Autodesk Inventor part; units mm, degrees
(part 2 of 2)
  spline S246 degree 2 poles (-6.4112, 55.0598) (-7.1438, 55.0598) (-8.0125, 55.9058) (-8.0125, 56.5866) knots 0 0 0 1 2 2 2
  spline S247 degree 2 poles (-8.0125, 56.5866) (-8.0125, 56.8945) (-7.8504, 57.3645) (-7.6786, 57.5428) knots 0 0 0 1 2 2 2
  spline S248 degree 2 poles (-7.6786, 57.5428) (-7.5068, 57.7211) (-7.0109, 57.9091) (-6.6511, 57.9091) knots 0 0 0 1 2 2 2
  line L247 (-6.6511, 57.9091) -> (-6.3755, 57.9091)
  line L248 (-6.3755, 57.9091) -> (-6.3755, 55.6238)
  spline S249 degree 2 poles (-6.3755, 55.6238) (-5.8537, 55.6238) (-5.2994, 56.2041) (-5.2994, 56.713) knots 0 0 0 1 2 2 2
  spline S250 degree 2 poles (-5.2994, 56.713) (-5.2994, 56.8977) (-5.3739, 57.2478) (-5.4323, 57.3905) knots 0 0 0 1 2 2 2
  spline S251 degree 2 poles (-5.4323, 57.3905) (-5.4971, 57.5396) (-5.6105, 57.747) (-5.6624, 57.8151) knots 0 0 0 1 2 2 2
  line L249 (-5.6624, 57.8151) -> (-5.6624, 57.8475)
  line L250 (-5.6624, 57.8475) -> (-5.1114, 57.8475)
  spline S252 degree 2 poles (-5.1114, 57.8475) (-5.0757, 57.7503) (-4.972, 57.4618) (-4.9428, 57.3451) knots 0 0 0 1 2 2 2
  spline S253 degree 2 poles (-4.9428, 57.3451) (-4.9007, 57.183) (-4.8585, 56.9204) (-4.8585, 56.7195) knots 0 0 0 1 2 2 2
  spline S254 degree 2 poles (-6.7613, 57.3678) (-6.9655, 57.3613) (-7.2637, 57.2673) (-7.3642, 57.1798) knots 0 0 0 1 2 2 2
  spline S255 degree 2 poles (-7.3642, 57.1798) (-7.4776, 57.0825) (-7.5976, 56.7778) (-7.5976, 56.5541) knots 0 0 0 1 2 2 2
  spline S256 degree 2 poles (-7.5976, 56.5541) (-7.5976, 56.3305) (-7.4776, 56.0225) (-7.361, 55.8961) knots 0 0 0 1 2 2 2
  spline S257 degree 2 poles (-7.361, 55.8961) (-7.241, 55.7729) (-6.9525, 55.64) (-6.7613, 55.6238) knots 0 0 0 1 2 2 2
  line L251 (-6.7613, 55.6238) -> (-6.7613, 57.3678)
  spline S258 degree 2 poles (-4.8585, 59.9026) (-4.8585, 59.1149) (-5.6657, 58.243) (-6.4112, 58.243) knots 0 0 0 1 2 2 2
  spline S259 degree 2 poles (-6.4112, 58.243) (-7.1438, 58.243) (-8.0125, 59.089) (-8.0125, 59.7697) knots 0 0 0 1 2 2 2
  spline S260 degree 2 poles (-8.0125, 59.7697) (-8.0125, 60.0776) (-7.8504, 60.5477) (-7.6786, 60.7259) knots 0 0 0 1 2 2 2
  spline S261 degree 2 poles (-7.6786, 60.7259) (-7.5068, 60.9042) (-7.0109, 61.0922) (-6.6511, 61.0922) knots 0 0 0 1 2 2 2
  line L252 (-6.6511, 61.0922) -> (-6.3755, 61.0922)
  line L253 (-6.3755, 61.0922) -> (-6.3755, 58.807)
  spline S262 degree 2 poles (-6.3755, 58.807) (-5.8537, 58.807) (-5.2994, 59.3872) (-5.2994, 59.8961) knots 0 0 0 1 2 2 2
  spline S263 degree 2 poles (-5.2994, 59.8961) (-5.2994, 60.0809) (-5.3739, 60.431) (-5.4323, 60.5736) knots 0 0 0 1 2 2 2
  spline S264 degree 2 poles (-5.4323, 60.5736) (-5.4971, 60.7227) (-5.6105, 60.9302) (-5.6624, 60.9982) knots 0 0 0 1 2 2 2
  line L254 (-5.6624, 60.9982) -> (-5.6624, 61.0306)
  line L255 (-5.6624, 61.0306) -> (-5.1114, 61.0306)
  spline S265 degree 2 poles (-5.1114, 61.0306) (-5.0757, 60.9334) (-4.972, 60.6449) (-4.9428, 60.5282) knots 0 0 0 1 2 2 2
  spline S266 degree 2 poles (-4.9428, 60.5282) (-4.9007, 60.3661) (-4.8585, 60.1036) (-4.8585, 59.9026) knots 0 0 0 1 2 2 2
  spline S267 degree 2 poles (-6.7613, 60.5509) (-6.9655, 60.5444) (-7.2637, 60.4504) (-7.3642, 60.3629) knots 0 0 0 1 2 2 2
  spline S268 degree 2 poles (-7.3642, 60.3629) (-7.4776, 60.2657) (-7.5976, 59.961) (-7.5976, 59.7373) knots 0 0 0 1 2 2 2
  spline S269 degree 2 poles (-7.5976, 59.7373) (-7.5976, 59.5136) (-7.4776, 59.2057) (-7.361, 59.0793) knots 0 0 0 1 2 2 2
  spline S270 degree 2 poles (-7.361, 59.0793) (-7.241, 58.9561) (-6.9525, 58.8232) (-6.7613, 58.807) knots 0 0 0 1 2 2 2
  line L256 (-6.7613, 58.807) -> (-6.7613, 60.5509)
  line L257 (-7.3869, 63.4002) -> (-7.3869, 63.371)
  spline S271 degree 2 poles (-7.3869, 63.371) (-7.4031, 63.3094) (-7.4096, 63.17) (-7.4096, 63.0728) knots 0 0 0 1 2 2 2
  spline S272 degree 2 poles (-7.4096, 63.0728) (-7.4096, 62.8491) (-7.2313, 62.405) (-7.0563, 62.2073) knots 0 0 0 1 2 2 2
  line L258 (-7.0563, 62.2073) -> (-4.9266, 62.2073)
  line L259 (-4.9266, 62.2073) -> (-4.9266, 61.653)
  line L260 (-4.9266, 61.653) -> (-7.9282, 61.653)
  line L261 (-7.9282, 61.653) -> (-7.9282, 62.2073)
  line L262 (-7.9282, 62.2073) -> (-7.4809, 62.2073)
  spline S273 degree 2 poles (-7.4809, 62.2073) (-7.7272, 62.512) (-7.9282, 62.9626) (-7.9282, 63.1765) knots 0 0 0 1 2 2 2
  spline S274 degree 2 poles (-7.9282, 63.1765) (-7.9282, 63.2608) (-7.9217, 63.3483) (-7.912, 63.4002) knots 0 0 0 1 2 2 2
  line L263 (-7.912, 63.4002) -> (-7.3869, 63.4002)
  line L264 (-4.9266, 64.3953) -> (-4.9266, 63.841)
  line L265 (-4.9266, 63.841) -> (-7.9282, 63.841)
  line L266 (-7.9282, 63.841) -> (-7.9282, 64.3953)
  line L267 (-7.9282, 64.3953) -> (-4.9266, 64.3953)
  line L268 (-8.4274, 64.4375) -> (-8.4274, 63.8054)
  line L269 (-8.4274, 63.8054) -> (-8.9525, 63.8054)
  line L270 (-8.9525, 63.8054) -> (-8.9525, 64.4375)
  line L271 (-8.9525, 64.4375) -> (-8.4274, 64.4375)
  line L272 (-4.9266, 67.8054) -> (-4.9266, 67.2511)
  line L273 (-4.9266, 67.2511) -> (-6.6381, 67.2511)
  spline S275 degree 2 poles (-6.6381, 67.2511) (-6.8456, 67.2511) (-7.2021, 67.2057) (-7.3091, 67.1441) knots 0 0 0 1 2 2 2
  spline S276 degree 2 poles (-7.3091, 67.1441) (-7.4225, 67.076) (-7.5328, 66.8329) (-7.5328, 66.6255) knots 0 0 0 1 2 2 2
  spline S277 degree 2 poles (-7.5328, 66.6255) (-7.5328, 66.418) (-7.3318, 65.9772) (-7.1697, 65.7665) knots 0 0 0 1 2 2 2
  line L274 (-7.1697, 65.7665) -> (-4.9266, 65.7665)
  line L275 (-4.9266, 65.7665) -> (-4.9266, 65.2122)
  line L276 (-4.9266, 65.2122) -> (-7.9282, 65.2122)
  line L277 (-7.9282, 65.2122) -> (-7.9282, 65.7665)
  line L278 (-7.9282, 65.7665) -> (-7.5943, 65.7665)
  spline S278 degree 2 poles (-7.5943, 65.7665) (-7.7986, 66.0161) (-8.0125, 66.499) (-8.0125, 66.7681) knots 0 0 0 1 2 2 2
  spline S279 degree 2 poles (-8.0125, 66.7681) (-8.0125, 67.2543) (-7.429, 67.8054) (-6.8747, 67.8054) knots 0 0 0 1 2 2 2
  line L279 (-6.8747, 67.8054) -> (-4.9266, 67.8054)
  spline S280 degree 2 poles (-4.4469, 68.7065) (-4.4242, 68.7616) (-4.3528, 68.982) (-4.3237, 69.1182) knots 0 0 0 1 2 2 2
  spline S281 degree 2 poles (-4.3237, 69.1182) (-4.288, 69.2738) (-4.2459, 69.5331) (-4.2459, 69.6854) knots 0 0 0 1 2 2 2
  spline S282 degree 2 poles (-4.2459, 69.6854) (-4.2459, 69.9415) (-4.3691, 70.2981) (-4.4793, 70.3986) knots 0 0 0 1 2 2 2
  spline S283 degree 2 poles (-4.4793, 70.3986) (-4.5895, 70.4926) (-4.878, 70.5704) (-5.0627, 70.5704) knots 0 0 0 1 2 2 2
  line L280 (-5.0627, 70.5704) -> (-5.3253, 70.5704)
  spline S284 degree 2 poles (-5.3253, 70.5704) (-5.147, 70.3467) (-4.9785, 69.9156) (-4.9785, 69.5914) knots 0 0 0 1 2 2 2
  spline S285 degree 2 poles (-4.9785, 69.5914) (-4.9785, 69.0274) (-5.7402, 68.3597) (-6.4566, 68.3597) knots 0 0 0 1 2 2 2
  spline S286 degree 2 poles (-6.4566, 68.3597) (-6.8293, 68.3597) (-7.4063, 68.5898) (-7.6105, 68.7843) knots 0 0 0 1 2 2 2
  spline S287 degree 2 poles (-7.6105, 68.7843) (-7.8018, 68.9691) (-8.0125, 69.478) (-8.0125, 69.7503) knots 0 0 0 1 2 2 2
  spline S288 degree 2 poles (-8.0125, 69.7503) (-8.0125, 70.0063) (-7.9023, 70.3823) (-7.8018, 70.5704) knots 0 0 0 1 2 2 2
  line L281 (-7.8018, 70.5704) -> (-7.9282, 70.6028)
  line L282 (-7.9282, 70.6028) -> (-7.9282, 71.1246)
  line L283 (-7.9282, 71.1246) -> (-5.2702, 71.1246)
  spline S289 degree 2 poles (-5.2702, 71.1246) (-4.5052, 71.1246) (-3.7921, 70.3921) (-3.7921, 69.64) knots 0 0 0 1 2 2 2
  spline S290 degree 2 poles (-3.7921, 69.64) (-3.7921, 69.4002) (-3.8634, 68.8945) (-3.9217, 68.6773) knots 0 0 0 1 2 2 2
  line L284 (-3.9217, 68.6773) -> (-4.4469, 68.6773)
  line L285 (-4.4469, 68.6773) -> (-4.4469, 68.7065)
  line L286 (-5.7402, 70.5704) -> (-7.3901, 70.5704)
  spline S291 degree 2 poles (-7.3901, 70.5704) (-7.4809, 70.3629) (-7.5587, 70.0128) (-7.5587, 69.8378) knots 0 0 0 1 2 2 2
  spline S292 degree 2 poles (-7.5587, 69.8378) (-7.5587, 69.4164) (-6.9947, 68.9334) (-6.4663, 68.9334) knots 0 0 0 1 2 2 2
  spline S293 degree 2 poles (-6.4663, 68.9334) (-5.9671, 68.9334) (-5.4452, 69.3029) (-5.4452, 69.7146) knots 0 0 0 1 2 2 2
  spline S294 degree 2 poles (-5.4452, 69.7146) (-5.4452, 69.9318) (-5.6008, 70.3888) (-5.7402, 70.5704) knots 0 0 0 1 2 2 2
  point P0 (0, 0)
  constraints: 4 other
emboss "凸雕3" sketch "草图12" operation cut depth 1 direction (0, -1, 0)
